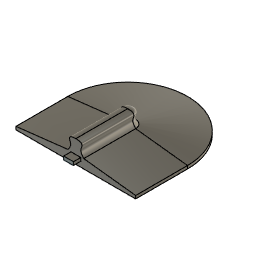
tanklid (Autodesk Fusion 360 design; units mm, degrees)
Autodesk Fusion 360 part; units mm, degrees
sketch "Skizze1" plane through (0, 0, 0) normal (0, 1, 0) x (1, 0, 0)
  line L0 (50, 0) -> (50, 2)
  line L1 (50, 2) -> (0, 2)
  line L2 (0, 2) -> (0, -19)
  line L3 (50, 0) -> (8, -6)
  line L4 (8, -6) -> (5, -11)
  arc A0 (5, -11) -> (5.4853, -14.3969) centre (7.3331, -12.3998) ccw
  arc A1 (4, -19) -> (5.4853, -14.3969) centre (3.6747, -16.3539) ccw
  line L5 (4, -19) -> (0, -19)
  constraint vertical L0
  constraint perpendicular L0 L1
  constraint perpendicular L1 L2
  constraint tangent L4 A0
  constraint tangent A0 A1
  constraint perpendicular L2 L5
sketch "Skizze2" plane through (0, 52, 0) normal (0, 1, 0) x (-1, 0, 0)
  line L0 (-50, 0) -> (-50, -2)
  line L1 (-50, -2) -> (50, -2)
  line L2 (50, -2) -> (50, 0)
  line L3 (50, 0) -> (8, 6)
  line L4 (8, 6) -> (5, 11)
  arc A0 (5.4853, 14.3969) -> (5, 11) centre (7.3331, 12.3998) ccw
  arc A1 (5.4853, 14.3969) -> (4, 19) centre (3.6747, 16.3539) ccw
  line L5 (4, 19) -> (-4, 19)
  arc A2 (-4, 19) -> (-5.4853, 14.3969) centre (-3.6747, 16.3539) ccw
  arc A3 (-5, 11) -> (-5.4853, 14.3969) centre (-7.3331, 12.3998) ccw
  line L6 (-5, 11) -> (-8, 6)
  line L7 (-8, 6) -> (-50, 0)
  line L8 (0, 2.5) -> (5, 2.5)
  line L9 (5, 2.5) -> (5, 6.5)
  line L10 (5, 6.5) -> (0, 6.5)
  line L11 (-5, 6.5) -> (0, 6.5)
  line L12 (-5, 2.5) -> (-5, 6.5)
  line L13 (0, 2.5) -> (-5, 2.5)
  constraint horizontal L8
  constraint vertical L9
  constraint horizontal L10
sketch "Skizze3" plane through (0, 0, -2) normal (0, 0, -1) x (1, 0, 0)
  line L0 (-50, 0) -> (-50, -52)
  line L1 (-50, -52) -> (50, -52)
  line L2 (50, -52) -> (50, 0)
  line L3 (42, -52) -> (42, 0)
  arc A0 (42, 0) -> (-42, 0) centre (0, 0) ccw
  line L4 (-42, 0) -> (-42, -52)
  line L5 (42, -52) -> (42, -35)
  line L6 (42, -35) -> (42, 0)
  line L7 (42, -35) -> (42, 0)
  line L8 (-42, 0) -> (0, 0)
  line L9 (0, 0) -> (36.3731, 21)
  line L10 (0, 0) -> (42, 0) construction
  line L11 (0, 0) -> (21, 36.3731)
  line L12 (0, 0) -> (42, 0) construction
  line L13 (0, 0) -> (0, 42)
  line L14 (0, 0) -> (-21, 36.3731)
  line L15 (0, 0) -> (42, 0) construction
  line L16 (0, 0) -> (-36.3731, 21)
  line L17 (0, 0) -> (42, 0) construction
  line L18 (-42, -52) -> (-42, -35)
  line L19 (50, 0) -> (-50, 0)
  dimension "d7" = 17
  dimension "d8" = 30
  dimension "d9" = 60
  dimension "d11" = 120
  dimension "d12" = 150
  dimension "d13" = 17
  constraint coincident L3 L5.end
  constraint coincident A0.centre L8.end
  constraint perpendicular L4 L8
  constraint horizontal L10
  constraint horizontal L12
  constraint coincident A0 L11.end
  constraint midpoint A0 L13.end
  constraint horizontal L15
  constraint coincident A0 L14.end
  constraint horizontal L17
  constraint perpendicular L1 L18
  constraint parallel L2 L3
  constraint parallel L0 L4
  constraint tangent L3 A0
  constraint tangent A0 L4
  measures "d7" distance of L3.start L5.end
  measures "d8" angle of L9 L10
  measures "d9" angle of L11 L12
  measures "d11" angle of L14 L15
  measures "d12" angle of L16 L17
  measures "d13" distance of L4.end L18.end
sketch "Skizze4" plane through (0, 0, -2) normal (0, 0, -1) x (1, 0, 0)
sketch "Skizze5" plane through (0, 0, 19) normal (0, 0, 1) x (-1, 0, 0)
  line L0 (-4, 0) -> (-4, -52)
  line L1 (-4, -52) -> (4, -52)
  line L2 (4, -52) -> (4, 0)
  line L3 (4, 0) -> (-4, 0)
sketch "Skizze6" plane through (0, 0, -2) normal (0, 0, -1) x (1, 0, 0)
  circle A0 centre (-42, -35) radius 5
  circle A1 centre (42, -35) radius 5
  line L0 (-50, 0) -> (-50, -52)
  line L1 (-50, -52) -> (50, -52)
  line L2 (50, -52) -> (50, 0)
  line L3 (-36.3731, 21) -> (0, 0)
  line L4 (-36.3731, 21) -> (-33.3731, 26.1962)
  line L5 (-36.3731, 21) -> (-39.3731, 15.8038)
  ellipse E0 centre (-36.3731, 21) end of major axis (-33.3731, 26.1962) minor radius 5.5
  line L6 (-39.3731, 15.8038) -> (-33.3731, 26.1962)
  line L7 (-31.6099, 18.25) -> (-41.1362, 23.75)
  line L8 (0, 0) -> (-21, 36.3731)
  line L9 (-21, 36.3731) -> (-26.1962, 33.3731)
  ellipse E1 centre (-21, 36.3731) end of major axis (-26.1962, 33.3731) minor radius 5.5
  line L10 (-15.8038, 39.3731) -> (-26.1962, 33.3731)
  line L11 (-23.75, 41.1362) -> (-18.25, 31.6099)
  line L12 (0, 42) -> (-6, 42)
  ellipse E2 centre (0, 42) end of major axis (-6, 42) minor radius 5.5
  line L13 (6, 42) -> (-6, 42)
  line L14 (0, 47.5) -> (0, 36.5)
  spline S0 degree 3 poles (-39.6231, 15.3708) (-38.1333, 14.5107) (-36.2374, 14.3955) (-34.5728, 15.0466) (-32.8594, 15.7167) (-31.4167, 17.181) (-30.7244, 18.9379) (-30.0525, 20.6429) (-30.0963, 22.6) (-30.8593, 24.1764) (-31.5855, 25.677) (-32.9561, 26.8056) (-34.5492, 27.2066) (-36.2418, 27.6327) (-38.1487, 27.2295) (-39.6338, 26.1534) (-41.1439, 25.0592) (-42.1983, 23.2895) (-42.4438, 21.4381) (-42.678, 19.6728) (-42.1721, 17.8567) (-41.0672, 16.5703) (-40.6558, 16.0912) (-40.1664, 15.6845) (-39.6231, 15.3708) knots -3.141593 -3.141593 -3.141593 -3.141593 -2.287952 -2.287952 -2.287952 -1.40931 -1.40931 -1.40931 -0.556686 -0.556686 -0.556686 0.254943 0.254943 0.254943 1.11731 1.11731 1.11731 1.994176 1.994176 1.994176 2.830265 2.830265 2.830265 3.141593 3.141593 3.141593 3.141593
  line L15 (0, 0) -> (21, 36.3731)
  line L16 (21, 36.3731) -> (15.8038, 39.3731)
  ellipse E3 centre (21, 36.3731) end of major axis (15.8038, 39.3731) minor radius 5.5
  line L17 (26.1962, 33.3731) -> (15.8038, 39.3731)
  line L18 (23.75, 41.1362) -> (18.25, 31.6099)
  line L19 (0, 0) -> (36.3731, 21)
  line L20 (36.3731, 21) -> (39.3731, 15.8038)
  ellipse E4 centre (36.3731, 21) end of major axis (39.3731, 15.8038) minor radius 5.5
  line L21 (33.3731, 26.1962) -> (39.3731, 15.8038)
  line L22 (31.6099, 18.25) -> (41.1362, 23.75)
  line L23 (-42, 0) -> (-42, 6)
  ellipse E5 centre (-42, 0) end of major axis (-42, 6) minor radius 5.5
  line L24 (-42, -6) -> (-42, 6)
  line L25 (-36.5, 0) -> (-47.5, 0)
  line L26 (-42, 0) -> (-42, 6)
  ellipse E6 centre (-42, 0) end of major axis (-42, 6) minor radius 5.5
  line L27 (-42, -6) -> (-42, 6)
  line L28 (-36.5, 0) -> (-47.5, 0)
  line L29 (42, -35) -> (42, -29)
  ellipse E7 centre (42, -35) end of major axis (42, -29) minor radius 5.5
  line L30 (42, -41) -> (42, -29)
  line L31 (47.5, -35) -> (36.5, -35)
  line L32 (-42, -35) -> (-42, -29)
  ellipse E8 centre (-42, -35) end of major axis (-42, -29) minor radius 5.5
  line L33 (-42, -41) -> (-42, -29)
  line L34 (-36.5, -35) -> (-47.5, -35)
  spline S1 degree 3 poles (-42, -41.5) (-40.2798, -41.5) (-38.5803, -40.6518) (-37.4642, -39.2557) (-36.3155, -37.8186) (-35.7981, -35.8292) (-36.077, -33.9614) (-36.3477, -32.149) (-37.3642, -30.476) (-38.8131, -29.4923) (-40.1923, -28.5559) (-41.9436, -28.2638) (-43.5238, -28.713) (-45.2027, -29.1903) (-46.6525, -30.4929) (-47.4006, -32.1674) (-48.1613, -33.8701) (-48.1895, -35.9298) (-47.4765, -37.656) (-46.7966, -39.3018) (-45.4505, -40.6216) (-43.8504, -41.1833) (-43.2546, -41.3925) (-42.6274, -41.5) (-42, -41.5) knots -3.141593 -3.141593 -3.141593 -3.141593 -2.287952 -2.287952 -2.287952 -1.40931 -1.40931 -1.40931 -0.556686 -0.556686 -0.556686 0.254943 0.254943 0.254943 1.11731 1.11731 1.11731 1.994176 1.994176 1.994176 2.830265 2.830265 2.830265 3.141593 3.141593 3.141593 3.141593
  ellipse E9 centre (-21, 36.3731) end of major axis (-26.6292, 33.1231) minor radius 6
  ellipse E10 centre (0, 42) end of major axis (-6.5, 42) minor radius 6
  spline S2 degree 3 poles (26.6292, 33.1231) (27.4893, 34.6128) (27.6045, 36.5087) (26.9534, 38.1733) (26.2833, 39.8867) (24.819, 41.3295) (23.0621, 42.0218) (21.3571, 42.6936) (19.4, 42.6498) (17.8236, 41.8869) (16.323, 41.1606) (15.1944, 39.79) (14.7934, 38.1969) (14.3673, 36.5043) (14.7705, 34.5974) (15.8466, 33.1123) (16.9408, 31.6022) (18.7105, 30.5479) (20.5619, 30.3023) (22.3272, 30.0682) (24.1433, 30.5741) (25.4297, 31.6789) (25.9088, 32.0903) (26.3155, 32.5797) (26.6292, 33.1231) knots -3.141593 -3.141593 -3.141593 -3.141593 -2.287952 -2.287952 -2.287952 -1.40931 -1.40931 -1.40931 -0.556686 -0.556686 -0.556686 0.254943 0.254943 0.254943 1.11731 1.11731 1.11731 1.994176 1.994176 1.994176 2.830265 2.830265 2.830265 3.141593 3.141593 3.141593 3.141593
  ellipse E11 centre (36.3731, 21) end of major axis (39.6231, 15.3708) minor radius 6
  ellipse E12 centre (42, 0) end of major axis (42, 6.5) minor radius 6
  spline S3 degree 3 poles (42, -41.5) (43.7202, -41.5) (45.4197, -40.6518) (46.5358, -39.2557) (47.6845, -37.8186) (48.2019, -35.8292) (47.923, -33.9614) (47.6523, -32.149) (46.6358, -30.476) (45.1869, -29.4923) (43.8077, -28.5559) (42.0564, -28.2638) (40.4762, -28.713) (38.7973, -29.1903) (37.3475, -30.4929) (36.5994, -32.1674) (35.8387, -33.8701) (35.8105, -35.9298) (36.5235, -37.656) (37.2034, -39.3018) (38.5495, -40.6216) (40.1496, -41.1833) (40.7454, -41.3925) (41.3726, -41.5) (42, -41.5) knots -3.141593 -3.141593 -3.141593 -3.141593 -2.287952 -2.287952 -2.287952 -1.40931 -1.40931 -1.40931 -0.556686 -0.556686 -0.556686 0.254943 0.254943 0.254943 1.11731 1.11731 1.11731 1.994176 1.994176 1.994176 2.830265 2.830265 2.830265 3.141593 3.141593 3.141593 3.141593
  ellipse E13 centre (-42, 0) end of major axis (-42, 6.5) minor radius 6
  arc A2 (-2, 0) -> (2, 0) centre (0, 0) ccw
  line L35 (-2, 0) -> (-37, 0)
  arc A3 (-47, 0) -> (-37, 0) centre (-42, 0) ccw
  line L36 (-47, 0) -> (-50, 0)
  line L37 (50, 0) -> (47, 0)
  arc A4 (37, 0) -> (47, 0) centre (42, 0) ccw
  line L38 (37, 0) -> (2, 0)
  dimension "d20" = 6
  dimension "d21" = 6
  dimension "d22" = 11
  dimension "d23" = 6
  dimension "d24" = 11
  dimension "d25" = 11
  dimension "d26" = 0.5
  dimension "d27" = 6
  dimension "d28" = 11
  dimension "d29" = 6
  dimension "d30" = 11
  dimension "d31" = 11
  dimension "d32" = 11
  dimension "d33" = 11
  dimension "d34" = 11
  dimension "d35" = 0.5
  dimension "d38" = 0.5
  dimension "d39" = 6
  dimension "d40" = 0.5
  constraint coincident L3.end L8.start
  constraint perpendicular L3 L4
  constraint perpendicular L3 L5
  constraint coincident L3.start L4.start
  constraint coincident L5.end E0
  constraint coincident E0 L7.start
  constraint coincident E0 L7.end
  constraint perpendicular L8 L9
  constraint coincident L8.end L9.start
  constraint perpendicular L8 L10
  constraint coincident E1 L10.start
  constraint coincident L9.end E1
  constraint horizontal L12
  constraint coincident L12.start E2.centre
  constraint parallel L12 L13
  constraint coincident E2 L13.start
  constraint coincident L12.end E2
  constraint coincident E2 L14.start
  constraint coincident E2 L14.end
  constraint perpendicular L15 L16
  constraint coincident L15.end L16.start
  constraint perpendicular L15 L17
  constraint coincident E3 L17.start
  constraint coincident L16.end E3
  constraint perpendicular L19 L20
  constraint coincident L19.end L20.start
  constraint perpendicular L19 L21
  constraint coincident E4 L21.start
  constraint coincident L20.end E4
  constraint vertical L23
  constraint coincident L23.start E5.centre
  constraint parallel L23 L24
  constraint coincident E5 L24.start
  constraint coincident L23.end E5
  constraint coincident E5 L25.start
  constraint coincident E5 L25.end
  constraint vertical L26
  constraint parallel L26 L27
  constraint coincident E6 L24.start
  constraint coincident L23.end E6
  constraint coincident E6 L25.start
  constraint coincident E6 L25.end
  constraint coincident A1.centre L29.start
  constraint vertical L29
  constraint parallel L29 L30
  constraint coincident E7 L30.start
  constraint coincident L29.end E7
  constraint coincident E7 L31.start
  constraint coincident E7 L31.end
  constraint coincident A0.centre L32.start
  constraint vertical L32
  constraint parallel L32 L33
  constraint coincident E8 L33.start
  constraint coincident L32.end E8
  constraint coincident E8 L34.start
  constraint coincident E8 L34.end
  measures "d20" distance of L3.start L4.end
  measures "d21" distance of L3.start L5.end
  measures "d23" distance of L8.end L9.end
  measures "d27" distance of L15.end L16.end
  measures "d29" distance of L19.end L20.end
  measures "d39" distance of E6
sketch "Skizze7" plane through (0, 0, 19) normal (0, 0, 1) x (-1, 0, 0)
  line L0 (-4, 0) -> (-4, -52)
  line L1 (-4, -52) -> (4, -52)
  line L2 (4, -52) -> (4, 0)
  circle A0 centre (0, 0) radius 2
  arc A1 (-2, 0) -> (2, 0) centre (0, 0) ccw
  line L3 (-2, 0) -> (-4, 0)
  line L4 (4, 0) -> (2, 0)
  constraint coincident A0.centre A1.centre
sketch "Skizze8" plane through (0, 0, 0) normal (0, 0, 1) x (1, 0, 0)
sketch "Skizze9" plane through (0, 0, -3) normal (0, 0, -1) x (1, 0, 0)
  spline S0 degree 3 poles (42, -41.5) (41.3726, -41.5) (40.7454, -41.3925) (40.1496, -41.1833) (38.5495, -40.6216) (37.2034, -39.3018) (36.5235, -37.656) (35.8105, -35.9298) (35.8387, -33.8701) (36.5994, -32.1674) (37.3475, -30.4929) (38.7973, -29.1903) (40.4762, -28.713) (42.0564, -28.2638) (43.8077, -28.5559) (45.1869, -29.4923) (46.6358, -30.476) (47.6523, -32.149) (47.923, -33.9614) (48.2019, -35.8292) (47.6845, -37.8186) (46.5358, -39.2557) (45.4197, -40.6518) (43.7202, -41.5) (42, -41.5) knots -3.141593 -3.141593 -3.141593 -3.141593 -2.830265 -2.830265 -2.830265 -1.994176 -1.994176 -1.994176 -1.11731 -1.11731 -1.11731 -0.254943 -0.254943 -0.254943 0.556686 0.556686 0.556686 1.40931 1.40931 1.40931 2.287952 2.287952 2.287952 3.141593 3.141593 3.141593 3.141593
  spline S1 degree 3 poles (-42, -41.5) (-42.6274, -41.5) (-43.2546, -41.3925) (-43.8504, -41.1833) (-45.4505, -40.6216) (-46.7966, -39.3018) (-47.4765, -37.656) (-48.1895, -35.9298) (-48.1613, -33.8701) (-47.4006, -32.1674) (-46.6525, -30.4929) (-45.2027, -29.1903) (-43.5238, -28.713) (-41.9436, -28.2638) (-40.1923, -28.5559) (-38.8131, -29.4923) (-37.3642, -30.476) (-36.3477, -32.149) (-36.077, -33.9614) (-35.7981, -35.8292) (-36.3155, -37.8186) (-37.4642, -39.2557) (-38.5803, -40.6518) (-40.2798, -41.5) (-42, -41.5) knots -3.141593 -3.141593 -3.141593 -3.141593 -2.830265 -2.830265 -2.830265 -1.994176 -1.994176 -1.994176 -1.11731 -1.11731 -1.11731 -0.254943 -0.254943 -0.254943 0.556686 0.556686 0.556686 1.40931 1.40931 1.40931 2.287952 2.287952 2.287952 3.141593 3.141593 3.141593 3.141593
  line L0 (-50, 0) -> (-50, -52)
  line L1 (-50, -52) -> (50, -52)
  line L2 (50, -52) -> (50, 0)
  circle A0 centre (0, 0) radius 2
  ellipse E0 centre (42, 0) end of major axis (42, 6.5) minor radius 6 (36, 0) -> (48, 0) ccw
  line L3 (36, 0) -> (2, 0)
  arc A1 (-2, 0) -> (2, 0) centre (0, 0) ccw
  line L4 (-2, 0) -> (-36, 0)
  ellipse E1 centre (-42, 0) end of major axis (-42, 6.5) minor radius 6 (-48, 0) -> (-36, 0) ccw
  line L5 (-48, 0) -> (-50, 0)
  line L6 (50, 0) -> (48, 0)
  constraint coincident A0.centre A1.centre
sketch "Skizze10" plane through (0, 0, -3) normal (0, 0, -1) x (1, 0, 0)
  spline S0 degree 3 poles (42, -41.5) (41.3726, -41.5) (40.7454, -41.3925) (40.1496, -41.1833) (38.5495, -40.6216) (37.2034, -39.3018) (36.5235, -37.656) (35.8105, -35.9298) (35.8387, -33.8701) (36.5994, -32.1674) (37.3475, -30.4929) (38.7973, -29.1903) (40.4762, -28.713) (42.0564, -28.2638) (43.8077, -28.5559) (45.1869, -29.4923) (46.6358, -30.476) (47.6523, -32.149) (47.923, -33.9614) (48.2019, -35.8292) (47.6845, -37.8186) (46.5358, -39.2557) (45.4197, -40.6518) (43.7202, -41.5) (42, -41.5) knots -3.141593 -3.141593 -3.141593 -3.141593 -2.830265 -2.830265 -2.830265 -1.994176 -1.994176 -1.994176 -1.11731 -1.11731 -1.11731 -0.254943 -0.254943 -0.254943 0.556686 0.556686 0.556686 1.40931 1.40931 1.40931 2.287952 2.287952 2.287952 3.141593 3.141593 3.141593 3.141593
  spline S1 degree 3 poles (-42, -41.5) (-42.6274, -41.5) (-43.2546, -41.3925) (-43.8504, -41.1833) (-45.4505, -40.6216) (-46.7966, -39.3018) (-47.4765, -37.656) (-48.1895, -35.9298) (-48.1613, -33.8701) (-47.4006, -32.1674) (-46.6525, -30.4929) (-45.2027, -29.1903) (-43.5238, -28.713) (-41.9436, -28.2638) (-40.1923, -28.5559) (-38.8131, -29.4923) (-37.3642, -30.476) (-36.3477, -32.149) (-36.077, -33.9614) (-35.7981, -35.8292) (-36.3155, -37.8186) (-37.4642, -39.2557) (-38.5803, -40.6518) (-40.2798, -41.5) (-42, -41.5) knots -3.141593 -3.141593 -3.141593 -3.141593 -2.830265 -2.830265 -2.830265 -1.994176 -1.994176 -1.994176 -1.11731 -1.11731 -1.11731 -0.254943 -0.254943 -0.254943 0.556686 0.556686 0.556686 1.40931 1.40931 1.40931 2.287952 2.287952 2.287952 3.141593 3.141593 3.141593 3.141593
  line L0 (-50, 0) -> (-50, -52)
  line L1 (-50, -52) -> (50, -52)
  line L2 (50, -52) -> (50, 0)
  ellipse E0 centre (42, 0) end of major axis (42, 6.5) minor radius 6 (36, 0) -> (48, 0) ccw
  line L3 (36, 0) -> (2, 0)
  arc A0 (-2, 0) -> (2, 0) centre (0, 0) ccw
  line L4 (-2, 0) -> (-36, 0)
  ellipse E1 centre (-42, 0) end of major axis (-42, 6.5) minor radius 6 (-48, 0) -> (-36, 0) ccw
  line L5 (-48, 0) -> (-50, 0)
  line L6 (50, 0) -> (48, 0)
sketch "Skizze11" plane through (0, 52, 0) normal (0, 1, 0) x (-1, 0, 0) in component "Oben"
  line L0 (-50, -2) -> (-50, -3)
  line L1 (-50, -3) -> (50, -3)
  line L2 (50, -3) -> (50, -2)
  line L3 (0, -3) -> (60, -3)
  line L4 (60, -3) -> (60, 0)
  line L5 (60, 0) -> (8, 6)
  spline S0 degree 5 poles (8, 6) (7.8622, 6.1522) (7.5949, 6.455) (7.2185, 6.9049) (6.7658, 7.4959) (6.2822, 8.2195) (5.8815, 8.9271) (5.5634, 9.6167) (5.3273, 10.2853) (5.1716, 10.9287) (5.0934, 11.5407) (5.0879, 12.1145) (5.1486, 12.6462) (5.2663, 13.1369) (5.4292, 13.5958) (5.6219, 14.043) (5.826, 14.5026) (6.0205, 14.995) (6.1818, 15.5306) (6.2842, 16.0998) (6.3019, 16.6769) (6.213, 17.2294) (6.0031, 17.7256) (5.6692, 18.1437) (5.2223, 18.4783) (4.6826, 18.735) (4.0748, 18.9265) (3.4237, 19.068) (2.7489, 19.1722) (2.0632, 19.2474) (1.3743, 19.2987) (0.8237, 19.3227) (0.4115, 19.3316) (0.1371, 19.3334) (0, 19.3333) knots 0 0 0 0 0 0 0.033333 0.066667 0.1 0.133333 0.166667 0.2 0.233333 0.266667 0.3 0.333333 0.366667 0.4 0.433333 0.466667 0.5 0.533333 0.566667 0.6 0.633333 0.666667 0.7 0.733333 0.766667 0.8 0.833333 0.866667 0.9 0.933333 0.966667 1 1 1 1 1 1
  line L6 (0, 19.3333) -> (0, -3)
  line L7 (0, 19.3333) -> (0, -3)
  line L8 (0, 19.3333) -> (0, -3)
  line L9 (60, -3) -> (0, -3)
  line L10 (50, -2) -> (-50, -2)
  point P0 (5.2745, 10.5425)
  point P1 (5.2844, 13.152)
  point P2 (6.0701, 15.1836)
  point P3 (6.0067, 17.6459)
  point P4 (3.7079, 19)
  constraint midpoint L1 L3.start
  constraint perpendicular L2 L3
  constraint perpendicular L3 L4
  constraint coincident L5.end S0.start
  constraint perpendicular L1 L6
revolve "Drehen1" add sketch "Skizze11" angle 180 about axis through (0, 52, 19.3333) along (0, 0, -1) contours L1 L2 L3 L6 L7 L8 L9 L10 | L2 L3 L4 L5 S0 L6 L7 L8 L9 L10 makes body 1 in component "Oben"
extrude "Extrusion1" add 2 faces at (-19.3333, 52, 0) (19.3333, 52, 0) along direction (0, -1, 0) blind 52 on bodies 1 bodies 1 in component "Oben"
sketch "Skizze1 (2)" plane through (0, 0, -3) normal (0, 0, -1) x (1, 0, 0) in component "Oben"
  arc A0 (-60, -52) -> (60, -52) centre (0, -52) ccw
  line L0 (60, -52) -> (60, 0)
  line L1 (60, 0) -> (-60, 0)
  line L2 (-60, 0) -> (-60, -52)
  line L3 (0, -112) -> (0, -52)
  line L4 (0, -52) -> (-60, -52)
  line L5 (60, -52) -> (0, -52)
  line L6 (-52, 0) -> (-52, -52)
  arc A1 (-52, -52) -> (52, -52) centre (0, -52) ccw
  line L7 (52, -52) -> (52, 0)
  line L8 (-52, -52) -> (-52, -17)
  line L9 (52, -52) -> (52, -17)
  line L10 (52, -17) -> (52, -52)
  line L11 (-52, -52) -> (-52, -17)
  line L12 (52, -52) -> (52, -17)
  line L13 (0, -52) -> (45.0333, -78)
  line L14 (0, -52) -> (52, -52) construction
  line L15 (0, -52) -> (26, -97.0333)
  line L16 (0, -52) -> (52, -52) construction
  line L17 (0, -52) -> (-26, -97.0333)
  line L18 (0, -52) -> (52, -52) construction
  line L19 (0, -52) -> (-45.0333, -78)
  line L20 (0, -52) -> (52, -52) construction
  line L21 (0, -52) -> (0, -104)
  dimension "d66" = -8
  dimension "d67" = 35
  dimension "d68" = 35
  dimension "d69" = 30
  dimension "d70" = 60
  dimension "d71" = 120
  dimension "d72" = 150
  constraint midpoint A0 L3.start
  constraint coincident A0.centre L3.end
  constraint coincident A0.start L2.end
  constraint coincident A0.end L0.start
  constraint coincident L6 L8.end
  constraint perpendicular L4 L8
  constraint coincident L7 L9.end
  constraint perpendicular L5 L9
  constraint perpendicular L4 L11
  constraint perpendicular L5 L12
  constraint horizontal L14
  constraint horizontal L16
  constraint horizontal L18
  constraint horizontal L20
  constraint coincident A1 L19.end
  constraint vertical L21
  measures "d67" distance of L6.end L8.end
  measures "d68" distance of A1.end L9.end
  measures "d69" angle of L13 L14
  measures "d70" angle of L15 L16
  measures "d71" angle of L17 L18
  measures "d72" angle of L19 L20
hole "Bohrung1" at (-52, 17, -3) at (-52, 52, -3) at (-45.0333, 78, -3) at (-26, 97.0333, -3) at (0, 104, -3) at (26, 97.0333, -3) at (45.0333, 78, -3) at (52, 52, -3) at (52, 17, -3) direction (0, 0, 1) diameter 10.5 depth 2 tip angle 180 bodies 1 in component "Oben"
sketch "Skizze2 (2)" plane through (0, 0, 0) normal (0, -1, 0) x (1, 0, 0) in component "Oben"
  line L0 (-8, 6) -> (-60, 0)
  line L1 (-60, 0) -> (-60, -3)
  line L2 (-60, -3) -> (60, -3)
  line L3 (60, -3) -> (60, 0)
  line L4 (60, 0) -> (8, 6)
  spline S0 degree 5 poles (8, 6) (7.8622, 6.1522) (7.5949, 6.455) (7.2185, 6.9049) (6.7658, 7.4959) (6.2822, 8.2195) (5.8815, 8.9271) (5.5634, 9.6167) (5.3273, 10.2853) (5.1716, 10.9287) (5.0934, 11.5407) (5.0879, 12.1145) (5.1486, 12.6462) (5.2663, 13.1369) (5.4292, 13.5958) (5.6219, 14.043) (5.826, 14.5026) (6.0205, 14.995) (6.1818, 15.5306) (6.2842, 16.0998) (6.3019, 16.6769) (6.213, 17.2294) (6.0031, 17.7256) (5.6692, 18.1437) (5.2223, 18.4783) (4.6826, 18.735) (4.0748, 18.9265) (3.4237, 19.068) (2.7489, 19.1722) (2.0632, 19.2474) (1.3743, 19.2987) (0.8237, 19.3227) (0.4115, 19.3316) (0.1371, 19.3334) (0, 19.3333) knots 0 0 0 0 0 0 0.033333 0.066667 0.1 0.133333 0.166667 0.2 0.233333 0.266667 0.3 0.333333 0.366667 0.4 0.433333 0.466667 0.5 0.533333 0.566667 0.6 0.633333 0.666667 0.7 0.733333 0.766667 0.8 0.833333 0.866667 0.9 0.933333 0.966667 1 1 1 1 1 1
  line L5 (0, -3) -> (0, 2)
  line L6 (0, 2) -> (-5, 2)
  line L7 (-5, 2) -> (-5, 5.5)
  line L8 (-5, 5.5) -> (5, 5.5)
  line L9 (5, 5.5) -> (5, 2)
  line L10 (5, 2) -> (0, 2)
  spline S1 degree 5 poles (0, 19.3333) (-0.1371, 19.3334) (-0.4115, 19.3316) (-0.8237, 19.3227) (-1.3743, 19.2987) (-2.0632, 19.2474) (-2.7489, 19.1722) (-3.4237, 19.068) (-4.0748, 18.9265) (-4.6826, 18.735) (-5.2223, 18.4783) (-5.6692, 18.1437) (-6.0031, 17.7256) (-6.213, 17.2294) (-6.3019, 16.6769) (-6.2842, 16.0998) (-6.1818, 15.5306) (-6.0205, 14.995) (-5.826, 14.5026) (-5.6219, 14.043) (-5.4292, 13.5958) (-5.2663, 13.1369) (-5.1486, 12.6462) (-5.0879, 12.1145) (-5.0934, 11.5407) (-5.1716, 10.9287) (-5.3273, 10.2853) (-5.5634, 9.6167) (-5.8815, 8.9271) (-6.2822, 8.2195) (-6.7658, 7.4959) (-7.2185, 6.9049) (-7.5949, 6.455) (-7.8622, 6.1522) (-8, 6) knots -1 -1 -1 -1 -1 -1 -0.966667 -0.933333 -0.9 -0.866667 -0.833333 -0.8 -0.766667 -0.733333 -0.7 -0.666667 -0.633333 -0.6 -0.566667 -0.533333 -0.5 -0.466667 -0.433333 -0.4 -0.366667 -0.333333 -0.3 -0.266667 -0.233333 -0.2 -0.166667 -0.133333 -0.1 -0.066667 -0.033333 0 0 0 0 0 0
  constraint midpoint L2 L5.start
  constraint perpendicular L2 L5
  constraint perpendicular L5 L6
  constraint perpendicular L6 L7
  constraint perpendicular L5 L8
  constraint perpendicular L6 L9
  constraint perpendicular L5 L10
extrude "Extrusion2" cut sketch "Skizze2 (2)" against normal blind 7.5 contours L6 L7 L8 L9 L10 bodies 1 in component "Oben"
sketch "Skizze1 (3)" plane through (0, 7.5, 0) normal (0, -1, 0) x (1, 0, 0) in component "Verbinder"
sketch "Skizze2 (3)" plane through (0, 7.5, 3.75) normal (0, -1, 0) x (1, 0, 0) in component "Verbinder"
sketch "Skizze3 (2)" plane through (0, 0, 0) normal (0, -1, 0) x (1, 0, 0) in component "Verbinder"
  line L0 (-5, 5.5) -> (5, 5.5)
  line L1 (5, 5.5) -> (5, 2)
  line L2 (5, 2) -> (-5, 2)
  line L3 (-5, 2) -> (-5, 5.5)
  line L4 (4.8, 2.2) -> (-4.8, 2.2)
  line L5 (-4.8, 2.2) -> (-4.8, 5.3)
  line L6 (-4.8, 5.3) -> (4.8, 5.3)
  line L7 (4.8, 5.3) -> (4.8, 2.2)
  dimension "d79" = 0.2
  constraint horizontal L0
  constraint vertical L1
  constraint horizontal L2
  constraint vertical L3
extrude "Extrusion1'" add sketch "Skizze3 (2)" against normal blind 7.3 separate body contours L4 L5 L6 L7 makes body 2 in component "Verbinder"
extrude "Extrusion2'" add 1 faces at (-1.6, 0, 4.2667) along direction (0, -1, 0) blind 7.3 on bodies 2 bodies 2 in component "Verbinder"
sketch "Skizze6 (2)" plane through (0, -7.3, 0) normal (0, -1, 0) x (1, 0, 0) in component "Oben"
  line L0 (4.8, 5.3) -> (-4.8, 5.3)
  line L1 (-4.8, 5.3) -> (-4.8, 2.2)
  line L2 (-4.8, 2.2) -> (4.8, 2.2)
  line L3 (4.8, 2.2) -> (4.8, 5.3)
sketch "Skizze1 (4)" plane through (0, 0, -3) normal (0, 0, -1) x (1, 0, 0) in component "Unten"
  circle A0 centre (52, -52) radius 5.25
  circle A1 centre (26, -97.0333) radius 5.25
  circle A2 centre (-26, -97.0333) radius 5.25
  circle A3 centre (-52, -52) radius 5.25
  circle A4 centre (-52, -17) radius 5.25
  circle A5 centre (-45.0333, -78) radius 5.25
  circle A6 centre (0, -104) radius 5.25
  circle A7 centre (45.0333, -78) radius 5.25
  circle A8 centre (52, -17) radius 5.25
  arc A9 (-60, -52) -> (60, -52) centre (0, -52) ccw
  line L0 (60, -52) -> (60, 0)
  line L1 (60, 0) -> (-60, 0)
  line L2 (-60, 0) -> (-60, -52)
  line L3 (0, -112) -> (0, -52)
  circle A10 centre (0, -52) radius 32
  dimension "d84" = 64
  constraint midpoint A9 L3.start
  constraint coincident A9.centre L3.end
  measures "d84" diameter of A10
extrude "Extrusion1''" add sketch "Skizze1 (4)" along normal blind 11.5 separate body contours A10 makes body 3 in component "Unten"
sketch "Skizze7 (2)" plane through (0, 0, 0) normal (0, 0, 1) x (1, 0, 0) in component "Oben"
sketch "Skizze2 (4)" plane through (0, 0, 0) normal (0, 1, 0) x (1, 0, 0) in component "Unten"
sketch "Skizze3 (3)" plane through (0, 0, 0) normal (0, 0, 1) x (1, 0, 0) in component "Unten"
sketch "Skizze4 (2)" plane through (0, 0, 0) normal (0, 0, 1) x (1, 0, 0) in component "Unten"
sketch "Skizze5 (2)" plane through (0, 0, -3) normal (0, 0, 1) x (-1, 0, 0) in component "Unten"
  circle A0 centre (0, -52) radius 32
extrude "Extrusion2''" cut sketch "Skizze5 (2)" against normal blind 6.5 bodies 3 in component "Unten"
sketch "Skizze6 (3)" plane through (0, 0, -9.5) normal (0, 0, 1) x (-1, 0, 0) in component "Unten"
  circle A0 centre (0, -52) radius 32
  circle A1 centre (0, -52) radius 30.8
  dimension "d89" = -1.2
extrude "Extrusion3" add sketch "Skizze6 (3)" along normal blind 1 contours A1 bodies 3 in component "Unten"
extrude "Extrusion4" add 1 faces at (-3.4094, 37.8867, -8.5) along direction (0, 0, 1) blind 0.5 on bodies 3 bodies 3 in component "Unten"
sketch "Skizze7 (3)" plane through (0, 0, -8) normal (0, 0, 1) x (-1, 0, 0) in component "Unten"
  circle A0 centre (0, -52) radius 30.8
  circle A1 centre (0, -52) radius 32
  dimension "d94" = 1.2
extrude "Extrusion5" add sketch "Skizze7 (3)" along normal blind 5 contours A0 | A1 bodies 3 in component "Unten"
sketch "Skizze12" plane through (0, 0, -14.5) normal (0, 0, -1) x (1, 0, 0)
  circle A0 centre (0, -52) radius 32
  line L0 (0, -52) -> (32, -52)
  constraint coincident A0.centre L0.start
  constraint coincident A0 L0.end
  constraint horizontal L0
sketch "Skizze13" plane through (0, 0, -14.5) normal (0, 0, -1) x (1, 0, 0)
  circle A0 centre (0, -52) radius 32
  line L0 (0, -52) -> (0, -20)
  line L1 (0, -52) -> (32, -52)
  line L2 (0, -52) -> (-20.4865, -76.5825)
  constraint coincident A0.centre L0.start
  constraint coincident A0 L0.end
  constraint vertical L0
  constraint coincident A0 L1.end
  constraint perpendicular L0 L1
  constraint coincident A0 L2.end
sketch "Skizze14" plane through (0, 0, -14.5) normal (0, 0, -1) x (1, 0, 0)
  circle A0 centre (0, -52) radius 32
hole "Bohrung2" at (0, 52, -14.5) direction (0, 0, 1) diameter 5 depth 28 tip angle 118 counterbore diameter 10 counterbore depth 7 bodies 1 in component "Oben"
hole "Bohrung1'" at (0, 52, -14.5) direction (0, 0, 1) diameter 5 depth 28 tip angle 118 counterbore diameter 10 counterbore depth 7 bodies 3 in component "Unten"
extrude "Extrusion3'" add 1 faces at (4.8, -2.4333, 4.2667) along direction (1, 0, 0) blind 0.1 on bodies 2 bodies 2 in component "Verbinder"
extrude "Extrusion4'" add 1 faces at (-1.5667, 2.4333, 5.3) along direction (0, 0, 1) blind 0.1 on bodies 2 bodies 2 in component "Verbinder"
extrude "Extrusion5'" add 1 faces at (-4.8, 2.4333, 4.3333) along direction (-1, 0, 0) blind 0.1 on bodies 2 bodies 2 in component "Verbinder"
extrude "Extrusion6" add 1 faces at (1.6333, -2.4333, 2.2) along direction (0, 0, -1) blind 0.1 on bodies 2 bodies 2 in component "Verbinder"
component "Oben" placed x (1, 0, 0) y (0, 1, 0) z (0, 0, 1) at (0, 0, 0)
component "Verbinder" placed x (1, 0, 0) y (0, 1, 0) z (0, 0, 1) at (0, 0, 0)
component "Unten" placed x (1, 0, 0) y (0, 1, 0) z (0, 0, 1) at (0, 0, 0)
